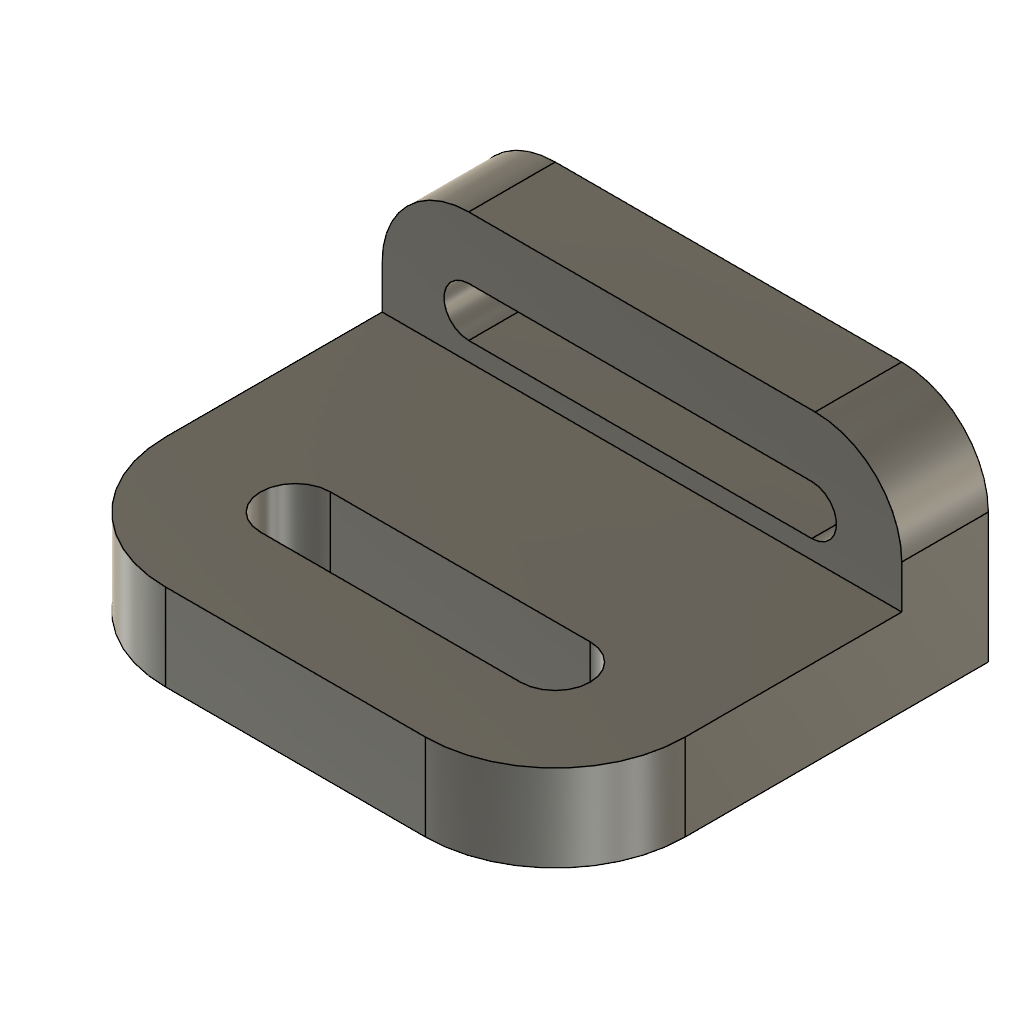
exercise 2 (Autodesk Fusion 360 design; units mm, degrees)
part number: 2026-10-01-22-08-37-260
Autodesk Fusion 360 part; units mm, degrees
sketch "Sketch1" plane through (0, 0, 0) normal (0, 1, 0) x (1, 0, 0)
  line L0 (-60, -10) -> (60, -10)
  line L1 (60, -10) -> (60, 10)
  line L2 (60, 10) -> (-60, 10)
  line L3 (-60, 10) -> (-60, -10)
  line L4 (-60, -10) -> (60, 10) construction
  line L5 (60, -10) -> (-60, 10) construction
  line L6 (-60, -10) -> (-60, -20)
  line L7 (-40, -40) -> (40, -40)
  line L8 (60, -20) -> (60, -10)
  line L9 (39.2131, -14.2951) -> (-40, -14.2951)
  arc A0 (-40, -14.2951) -> (-40, -25.7049) centre (-40, -20) ccw
  line L10 (-40, -25.7049) -> (39.2131, -25.7049)
  arc A1 (39.2131, -25.7049) -> (39.2131, -14.2951) centre (39.2131, -20) ccw
  line L11 (39.2131, -20) -> (-40, -20) construction
  arc A2 (-60, -20) -> (-40, -40) centre (-40, -20) ccw
  arc A3 (40, -40) -> (60, -20) centre (40, -20) ccw
  point P0 (-60, -40)
  point P1 (60, -40)
  point P2 (-0.3934, -20)
  dimension "d1" = 20
  dimension "d2" = 120
  dimension "d3" = 30
  dimension "d4" = 120
  dimension "d5" = 20
  dimension "d6" = 20
  dimension "d7" = 30
  constraint horizontal L0
  constraint perpendicular L0 L1
  constraint parallel L0 L2
  constraint parallel L1 L3
  constraint coincident L4 origin
  constraint coincident L5 origin
  constraint perpendicular L0 L6
  constraint perpendicular L6 L7
  constraint tangent L9 A0
  constraint tangent A0 L10
  constraint parallel L9 L10
  constraint tangent L10 A1
  constraint tangent L9 A1
  constraint horizontal L11
  constraint midpoint L11 P2
  constraint coincident P0 L6
  constraint coincident P0 L7
  constraint tangent L6 A2
  constraint tangent L7 A2
  constraint coincident P1 L7
  constraint coincident P1 L8
  constraint tangent L7 A3
  constraint tangent L8 A3
  measures "d1" distance of L0.start L2.end
  measures "d2" distance of L1.end L2.end
  measures "d5" radius of A2
  measures "d6" radius of A3
  measures "d7" distance of L2 A1.centre
extrude "Extrude1" add sketch "Sketch1" along normal blind 20
sketch "Sketch2" plane through (-60, 0, 0) normal (-1, 0, 0) x (0, -1, 0)
  line L0 (0, -10) -> (0, 20)
  line L1 (0, 20) -> (-20, 20)
  line L2 (-20, 20) -> (-20, -10)
  line L3 (-20, -10) -> (0, -10)
  line L4 (0, -10) -> (80, -10)
  line L5 (80, -10) -> (80, 10)
  line L6 (80, 10) -> (0, 10)
  line L7 (0, 10) -> (0, -10)
  dimension "d10" = 80
  dimension "d11" = 20
  constraint horizontal L4
  constraint vertical L5
  constraint horizontal L6
  constraint vertical L7
  constraint coincident L0.start L3.end
  measures "d10" distance of L0.start L4.end
  measures "d11" distance of L0.start L6.end
extrude "Extrude2" add sketch "Sketch2" against normal blind 120 contours L0 L4 L5 L6 L7
fillet "Fillet1" radius 30 2 edges at (-60, -80, 0) (60, -80, 0)
sketch "Sketch3" plane through (0, 0, 10) normal (0, 0, 1) x (-1, 0, 0)
  arc A0 (-30, 80) -> (-60, 50) centre (-30, 50) ccw
  line L0 (-60, 50) -> (-60, 0)
  line L1 (-60, 0) -> (60, 0)
  line L2 (60, 0) -> (60, 50)
  arc A1 (60, 50) -> (30, 80) centre (30, 50) ccw
  line L3 (30, 80) -> (-30, 80)
  line L4 (-30, 41.9438) -> (30, 41.9438)
  arc A2 (30, 41.9438) -> (30, 58.0562) centre (30, 50) ccw
  line L5 (30, 58.0562) -> (-30, 58.0562)
  arc A3 (-30, 58.0562) -> (-30, 41.9438) centre (-30, 50) ccw
  line L6 (-30, 50) -> (30, 50) construction
  point P0 (0, 50)
  dimension "d16" = 60
  dimension "d18" = 30
  constraint tangent L4 A2
  constraint tangent A2 L5
  constraint parallel L4 L5
  constraint tangent L5 A3
  constraint tangent L4 A3
  constraint parallel L1 L6
  constraint midpoint L6 P0
  measures "d5" radius of L5.end
  measures "d16" distance of A0.centre A1.centre
  measures "d18" distance of L2 A1.centre
extrude "Extrude3" cut sketch "Sketch3" against normal blind 58.307 contours L4 A2 L5 A3
